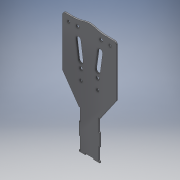
# Autodesk Inventor part: Arm - stand plate
Saved by Autodesk Inventor 2017 (Build 210142000, 142)
## iProperties
Created: 2016-08-03
Part Number: Arm - stand plate
Material: Generic
Document SubType Name: Modeling
Designer: Ali
Density: 1 g/cm^3
Appearance: Default
Author: Ali
Autodesk Inventor part; units mm, degrees
ref_plane "YZ Plane" through (0, 0, 0) normal (1, 0, 0) x (0, 1, 0)
ref_plane "XZ Plane" through (0, 0, 0) normal (0, 1, 0) x (-1, 0, 0)
ref_plane "XY Plane" through (0, 0, 0) normal (0, 0, 1) x (1, 0, 0)
sketch "Sketch1" plane through (0, 0, 0) normal (0, 0, 1) x (1, 0, 0)
  arc A0 (-20.3204, 17.9615) -> (-32.1264, 16.3566) centre (-26.2234, 17.159) ccw
  line L0 (-20.3204, 17.9615) -> (-14.6157, -24.0052)
  arc A1 (-26.4217, -25.6101) -> (-14.6157, -24.0052) centre (-20.5187, -24.8077) ccw
  line L1 (-26.4217, -25.6101) -> (-32.1264, 16.3566)
  arc A2 (-17.4681, 46.3619) -> (-13.8821, 37.9739) centre (-13.8821, 42.9344) ccw
  arc A3 (17.4681, 46.3619) -> (-17.4681, 46.3619) centre (0, 29.6659) ccw
  arc A4 (13.8821, 37.9739) -> (17.4681, 46.3619) centre (13.8821, 42.9344) ccw
  line L2 (13.8821, 37.9739) -> (-13.8821, 37.9739)
  arc A5 (32.1264, 16.3566) -> (20.3204, 17.9615) centre (26.2234, 17.159) ccw
  line L3 (32.1264, 16.3566) -> (26.4217, -25.6101)
  arc A6 (14.6157, -24.0052) -> (26.4217, -25.6101) centre (20.5187, -24.8077) ccw
  line L4 (14.6157, -24.0052) -> (20.3204, 17.9615)
  circle A7 centre (-28.3016, 42.9344) radius 4
  circle A8 centre (-20.018, -41.0528) radius 4
  circle A9 centre (20.018, -41.0528) radius 4
  circle A10 centre (28.3016, 42.9344) radius 4
  circle A11 centre (-50, 41.9238) radius 3.25
  circle A12 centre (50, 41.9238) radius 3.25
  circle A13 centre (20.018, -66.0762) radius 3.25
  circle A14 centre (-20.018, -66.0762) radius 3.25
  line L5 (64.7409, 50.3067) -> (64.7409, 34.44)
  arc A15 (64.7409, 50.3067) -> (58.7409, 56.3067) centre (58.7409, 50.3067) ccw
  line L6 (41.2562, 56.3067) -> (58.7409, 56.3067)
  arc A16 (12.5221, 61.0169) -> (41.2562, 56.3067) centre (41.2562, 146.3067) ccw
  arc A17 (12.5221, 61.0169) -> (-12.5221, 61.0169) centre (0, 23.8483) ccw
  arc A18 (-41.2562, 56.3067) -> (-12.5221, 61.0169) centre (-41.2562, 146.3067) ccw
  line L7 (-41.2562, 56.3067) -> (-58.7409, 56.3067)
  arc A19 (-58.7409, 56.3067) -> (-64.7409, 50.3067) centre (-58.7409, 50.3067) ccw
  line L8 (-64.7409, 50.3067) -> (-64.7409, 21.44)
  line L9 (-64.7409, 21.44) -> (-64.7409, -66.0762)
  line L10 (22, -123.1517) -> (25, -123.1517)
  line L11 (22, -153.1517) -> (25, -153.1517)
  line L12 (22, -183.1517) -> (25, -183.1517)
  line L13 (22, -213.1517) -> (25, -213.1517)
  line L14 (22, -183.1517) -> (22, -213.1517)
  line L15 (22, -123.1517) -> (22, -153.1517)
  line L16 (25, -153.1517) -> (25, -183.1517)
  line L17 (64.7409, -66.0762) -> (-64.7409, -66.0762) construction
  line L18 (64.7409, 34.44) -> (64.7409, -66.0762)
  line L19 (64.7409, -66.0762) -> (25, -123.1517)
  line L20 (25, -213.1517) -> (25, -216.1517)
  line L21 (25, -216.1517) -> (0, -216.1517)
  line L22 (0, -216.1517) -> (0, -66.0762)
  line L23 (-22, -123.1517) -> (-25, -123.1517)
  line L24 (-22, -153.1517) -> (-25, -153.1517)
  line L25 (-22, -183.1517) -> (-25, -183.1517)
  line L26 (-22, -213.1517) -> (-25, -213.1517)
  line L27 (-22, -183.1517) -> (-22, -213.1517)
  line L28 (-22, -123.1517) -> (-22, -153.1517)
  line L29 (-25, -153.1517) -> (-25, -183.1517)
  line L30 (-64.7409, -66.0762) -> (-25, -123.1517)
  line L31 (-25, -213.1517) -> (-25, -216.1517)
  line L32 (-25, -216.1517) -> (0, -216.1517)
  point P0 (20.018, -66.0762)
  point P1 (-64.7409, -22.3181)
  point P2 (27.0258, 23.062)
  point P3 (64.7409, 42.3734)
  dimension "d5" = 30
  dimension "d6" = 30
  dimension "d7" = 30
  dimension "d10" = 3
  dimension "d11" = 3
  dimension "d12" = 240
  dimension "d13" = 50
  constraints: 66 end point, 25 point on circle, 20 centre point, 9 symmetric about line, 6 point on line, 4 horizontal, 4 vertical, 3 midpoint, 2 parallel, 2 perpendicular, 1 collinear, 27 other
  measures "d5" distance between parallel lines of L11 L10
  measures "d6" distance between parallel lines of L12 L11
  measures "d7" distance between parallel lines of L12 L13
  measures "d10" distance between parallel lines of L15 L16
  measures "d11" distance of L13.end L20.end
  measures "d12" distance from line of A17.centre L32
  measures "d13" diameter of L29 L22
extrude "Extrusion1" add sketch "Sketch1" along normal blind 3 contours A3 A4 L2 A2 | L5 L18 L19 L10 L15 L11 L16 L12 L14 L13 L20 L21 L32 L31 L26 L27 L25 L29 L24 L28 L23 L30 L9 L8 A19 L7 A18 A17 A16 L6 A15
sketch "Sketch2" plane through (0, 0, 0) normal (0, 0, -1) x (-1, 0, 0)
  line L0 (-25, -216.1517) -> (25, -216.1517) projected
  line L1 (-10, -216.1517) -> (10, -216.1517)
  line L2 (10, -216.1517) -> (10, -213.1517)
  line L3 (10, -213.1517) -> (-10, -213.1517)
  line L4 (-10, -213.1517) -> (-10, -216.1517)
  line L5 (0, -213.1517) -> (0, -190.7997)
  point P0 (0, 0)
  dimension "d16" = 20
  dimension "d17" = 3
  constraints: 10 end point, 2 parallel, 2 point on line, 1 horizontal, 1 midpoint, 1 perpendicular, 1 vertical
  measures "d16" distance of L2.end L3.end
  measures "d17" distance between parallel lines of L0 L3
extrude "Extrusion2" cut sketch "Sketch2" against normal blind 6
body "Solid1"
